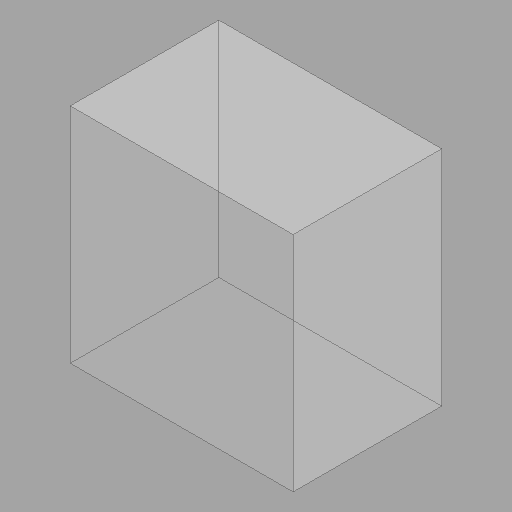
# Autodesk Inventor part: CE-7.1.1_CE-2.1.4_WP
Saved by Autodesk Inventor 2024 (Build 280153000, 153)
## iProperties
Created: 2024-02-25
Part Number: CE-7.1.1_CE-2.1.4_WP
Material: Generic
Document SubType Name: Modeling
Designer: Alex
Density: 1 g/cm^3
Appearance: Default
d0: -25.000 mm
d1: 37.500 mm
d2: 37.500 mm
d3: 37.500 mm
d4: 37.500 mm
d5: 50.000 mm
d6: 0.00 deg
Xmin: -37.500 mm
Ymin: -37.500 mm
Zmin: -25.000 mm
Xmax: 37.500 mm
Ymax: 37.500 mm
Zmax: 25.000 mm
Author: Alex
Autodesk Inventor part; units mm, degrees
ref_plane "YZ Plane" through (0, 0, 0) normal (1, 0, 0) x (0, 1, 0)
ref_plane "XZ Plane" through (0, 0, 0) normal (0, 1, 0) x (-1, 0, 0)
ref_plane "XY Plane" through (0, 0, 0) normal (0, 0, 1) x (1, 0, 0)
sketch "Sketch1" plane through (0, 0, -25) normal (0, 0, 1) x (1, 0, 0)
  line L0 (-37.5, 37.5) -> (37.5, 37.5)
  line L1 (37.5, 37.5) -> (37.5, -37.5)
  line L2 (37.5, -37.5) -> (-37.5, -37.5)
  line L3 (-37.5, -37.5) -> (-37.5, 37.5)
  point P0 (0, 0)
  dimension "d1" = 37.5
  dimension "d2" = 37.5
  dimension "d3" = 37.5
  dimension "d4" = 37.5
  constraints: 8 end point, 2 parallel, 1 horizontal, 1 perpendicular, 1 other
  measures "d1" distance from line of L3 point (0, 0)
  measures "d2" distance from line of L1 point (0, 0)
  measures "d3" distance from line of L2 point (0, 0)
  measures "d4" distance from line of L0 point (0, 0)
extrude "Extrusion1" add sketch "Sketch1" along normal blind 50
equation "\"d1\" = -Xmin"
equation "\"d2\" = Xmax"
equation "\"d3\" = -Ymin"
equation "\"d4\" = Ymax"
equation "\"d5\" = Zmax - Zmin"
equation "\"Xmin\" = -37.5"
equation "\"Ymin\" = -37.5"
equation "\"Zmin\" = -25"
equation "\"Xmax\" = 37.5"
equation "\"Ymax\" = 37.5"
equation "\"Zmax\" = 25"
body "Solid1"
